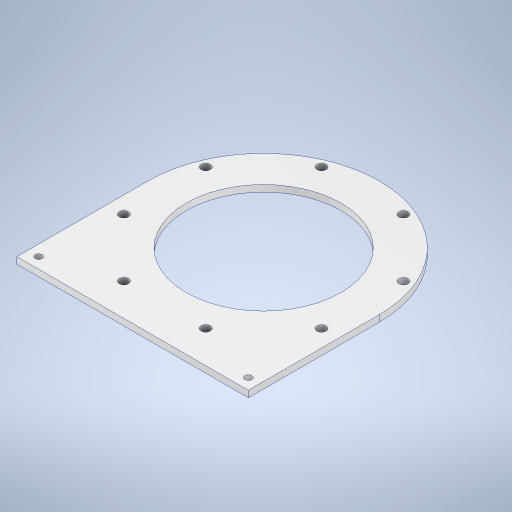
# Autodesk Inventor part: link2_plate1
Saved by Autodesk Inventor 2024 (Build 280153000, 153)
## iProperties
Created: 2024-12-13
Part Number: link2_plate1
Material: アルミニウム 6061
Document SubType Name: Sheet Metal
Designer: hirek
Density: 2.7 g/cm^3
Sheet Metal Rule: Default_mm
Appearance: アルミニウム - フラット
Author: hirek
Autodesk Inventor part; units mm, degrees
ref_plane "YZ Plane" through (0, 0, 0) normal (1, 0, 0) x (0, 1, 0)
ref_plane "XZ Plane" through (0, 0, 0) normal (0, 1, 0) x (-1, 0, 0)
ref_plane "XY Plane" through (0, 0, 0) normal (0, 0, 1) x (1, 0, 0)
sketch "スケッチ1" plane through (0, 0, 0) normal (0, 1, 0) x (-1, 0, 0)
  line L0 (0, 0) -> (106, 0)
  line L1 (106, 0) -> (106, -113)
  line L2 (106, -113) -> (0, -113)
  line L3 (0, -113) -> (0, 0)
  dimension "d0" = 106
  dimension "d1" = 113
  constraints: 8 end point, 2 parallel, 1 horizontal, 1 perpendicular
  measures "d0" distance of L1.end L2.end
  measures "d1" distance of L0.end L1.end
extrude "押し出し1" add sketch "スケッチ1" along normal blind 3
sketch "スケッチ3" plane through (0, 3, 0) normal (0, 1, 0) x (1, 0, 0)
  line L0 (-106, 113) -> (-106, 0) projected
  line L1 (0, 113) -> (-106, 113) projected
  circle A0 centre (-53, 60) radius 35.5
  line L2 (-106, 0) -> (0, 0) projected
  line L3 (-106, 60) -> (0, 60)
  line L4 (0, 0) -> (0, 113) projected
  circle A1 centre (-53, 60) radius 53
  point P0 (-53, 113)
  point P1 (0, 60)
  point P2 (-106, 60)
  dimension "d17" = 71
  dimension "d49" = 53
  dimension "d50" = 0
  dimension "d52" = 106
  constraints: 2 centre point, 2 end point, 2 point on line, 1 coincident, 1 horizontal, 1 midpoint
  measures "d17" diameter of A0
  measures "d49" distance between parallel lines of L3 L1
  measures "d50" distance of point (-53, 60) A0.centre
  measures "d52" diameter of A1
extrude "押し出し2" cut sketch "スケッチ3" against normal blind 3 contours L1 A1 L0 | L1 L4 A1 | L3 A0 | A0 L3
sketch "スケッチ4" plane through (0, 3, 0) normal (0, 1, 0) x (1, 0, 0)
  line L0 (-106, 113) -> (-106, 0) projected
  line L1 (-106, 5) -> (0, 5)
  line L2 (0, 0) -> (0, 113) projected
  line L3 (-106, 0) -> (0, 0) projected
  line L4 (0, 113) -> (-106, 113) projected
  line L5 (-106, 0) -> (0, 0) projected
  line L6 (-101, 0) -> (-101, 113)
  line L7 (-5, 113) -> (-5, 0)
  point P0 (-101, 5)
  point P1 (-5, 5)
  dimension "d22" = 5
  dimension "d24" = 5
  dimension "d25" = 5
  constraints: 10 point on line, 6 end point, 2 perpendicular, 1 horizontal
  measures "d22" distance between parallel lines of L1 L3
  measures "d24" distance between parallel lines of L0 L6
  measures "d25" distance between parallel lines of L2 L7
hole "穴2" at (-101, 3, -5) at (-5, 3, -5) direction (0, -1, 0) diameter 3.2 end through all
sketch "スケッチ5" plane through (0, 3, 0) normal (0, 1, 0) x (1, 0, 0)
  line L0 (-106, 113) -> (-106, 0) projected
  line L1 (-106, 60) -> (0, 60)
  circle A0 centre (-53, 60) radius 49
  line L2 (0, 113) -> (-106, 113) projected
  line L3 (-53, 60) -> (-7.7299, 78.7515)
  point P0 (0, 0)
  point P1 (-34.2485, 105.2701)
  point P2 (-71.7515, 105.2701)
  point P3 (-98.2701, 78.7515)
  point P4 (-98.2701, 41.2485)
  point P5 (-71.7515, 14.7299)
  point P6 (-34.2485, 14.7299)
  point P7 (-7.7299, 41.2485)
  dimension "d35" = 98
  dimension "d36" = 53
  dimension "d37" = 22.5
  dimension "d40" = 360
  constraints: 4 end point, 1 coincident, 1 midpoint, 1 perpendicular, 1 point on line, 12 other
  measures "d36" distance between parallel lines of L1 L2
  measures "d37" angle of L1 L3
hole "穴3" at (-7.7299, 3, -78.7515) at (-34.2485, 3, -105.2701) at (-71.7515, 3, -105.2701) at (-98.2701, 3, -78.7515) at (-98.2701, 3, -41.2485) at (-71.7515, 3, -14.7299) at (-34.2485, 3, -14.7299) at (-7.7299, 3, -41.2485) direction (0, -1, 0) diameter 4.2 end through all
equation "\"d47\" = Thickness"
equation "\"BendRadius\" = Thickness"
equation "\"BendReliefWidth\" = Thickness"
equation "\"BendReliefDepth\" = 0.5 * Thickness"
equation "\"CornerReliefSize\" = 4 * Thickness"
equation "\"MinimumRemnant\" = 2 * Thickness"
equation "\"TransitionRadius\" = BendRadius"
equation "\"JacobiRadiusSize\" = BendRadius"
equation "\"GapSize\" = Thickness"
equation "\"Thickness\" = 0.5"
